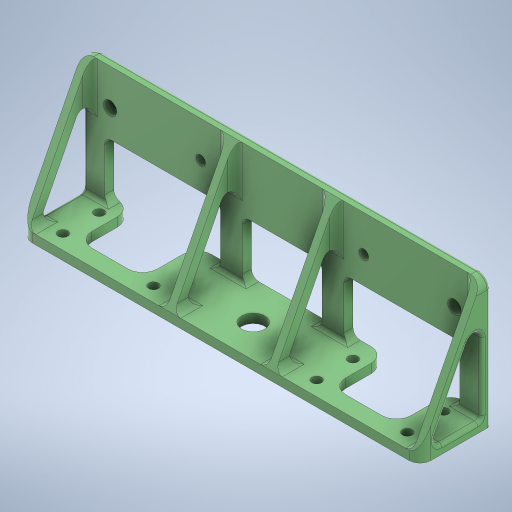
# Autodesk Inventor part: v3_realsense_mount
Saved by Autodesk Inventor 2024 (Build 280153000, 153)
## iProperties
Created: 2025-03-09
Part Number: v3_realsense_mount
Material: Generic
Document SubType Name: Modeling
Designer: Bruno
Density: 1 g/cm^3
Appearance: Default
Author: Bruno
Autodesk Inventor part; units mm, degrees
ref_plane "YZ Plane" through (0, 0, 0) normal (1, 0, 0) x (0, 1, 0)
ref_plane "XZ Plane" through (0, 0, 0) normal (0, 1, 0) x (-1, 0, 0)
sketch "Sketch1" plane through (0, 0, 0) normal (0, 1, 0) x (-1, 0, 0)
  line L0 (55, -9) -> (-55, -9)
  line L1 (-55, -9) -> (-55, 9)
  line L2 (-55, 9) -> (55, 9)
  line L3 (55, 9) -> (55, -9)
  line L4 (55, -9) -> (-55, 9)
  line L5 (55, 0) -> (-55, 0)
  line L6 (0, -9) -> (0, 9)
  circle A0 centre (0, 0) radius 3.2
  circle A1 centre (47.5, 5) radius 1.35
  circle A2 centre (22.5, 5) radius 1.35
  circle A3 centre (47.5, -5) radius 1.35
  circle A4 centre (22.5, -5) radius 1.35
  circle A5 centre (-47.5, 5) radius 1.35
  circle A6 centre (-22.5, 5) radius 1.35
  circle A7 centre (-47.5, -5) radius 1.35
  circle A8 centre (-22.5, -5) radius 1.35
  dimension "d0" = 18
  dimension "d1" = 110
  dimension "d2" = 6.4
  dimension "d3" = 2.7
  dimension "d4" = 2.7
  dimension "d5" = 45
  dimension "d6" = 95
  dimension "d7" = 10
  dimension "d8" = 10
  constraints: 14 end point, 9 centre point, 6 symmetric about line, 5 midpoint, 2 coincident, 2 parallel, 1 horizontal, 1 perpendicular, 6 other
  measures "d0" distance of L2.end L0.start
  measures "d1" distance of L1.end L2.end
  measures "d2" diameter of A0
  measures "d3" diameter of A1
  measures "d4" diameter of A2
  measures "d5" diameter of A2.centre L6
  measures "d6" diameter of A1.centre L6
  measures "d7" diameter of A2.centre L5
  measures "d8" diameter of A1.centre L5
extrude "Extrusion1" add sketch "Sketch1" along normal blind 2.5 contours L4 A4 A0 L5 L3 | L0 L6 A0 L4 A4 | L0 L1 L5 A0 L6 | L5 A0 L6 L2 L3 | L1 L4 A6 A0 L5 | L6 A0 L4 A6 L2
sketch "Sketch2" plane through (-55, 0, -9) normal (-1, 0, 0) x (0, 0, 1)
  line L0 (0, 0) -> (18, 0) projected
  line L1 (18, 0) -> (18, 2.5) projected
  line L2 (0, 2.5) -> (18, 2.5) projected
  line L3 (0, 0) -> (0, 2.5) projected
  line L4 (1, 0) -> (-1.5, 0)
  line L5 (-1.5, 0) -> (-1.5, 36)
  line L6 (-1.5, 36) -> (1, 36)
  line L7 (1, 36) -> (1, 0)
  point P0 (9, 0)
  point P1 (1, 2.5)
  dimension "d11" = 17
  dimension "d12" = 2.5
  dimension "d35" = 36
  constraints: 8 end point, 2 parallel, 1 horizontal, 1 perpendicular, 1 point on line
  measures "d11" distance between parallel lines of L7 L1
  measures "d12" distance of L5.end L6.end
  measures "d35" distance between parallel lines of L0 L6
extrude "Extrusion2" add sketch "Sketch2" against normal up to surface (110 mm away) contours L4 L5 L6 L7 L2 L3
sketch "Sketch3" plane through (-55, 2.5, -8) normal (0, 0, 1) x (1, 0, 0)
  line L0 (0, 33.5) -> (110, 33.5) projected
  line L1 (0, 0) -> (0, 33.5) projected
  line L2 (110, 0) -> (110, 33.5) projected
  line L3 (0, 23.5) -> (110, 23.5)
  circle A0 centre (7.5, 23.5) radius 1.85
  circle A1 centre (32.5, 23.5) radius 1.35
  line L4 (55, 33.5) -> (55, 1.216)
  circle A2 centre (102.5, 23.5) radius 1.85
  circle A3 centre (77.5, 23.5) radius 1.35
  line L5 (6, 16) -> (38, 16)
  line L6 (38, 16) -> (38, 0)
  line L7 (38, 0) -> (6, 0)
  line L8 (6, 0) -> (6, 16)
  line L9 (44, 16) -> (66, 16)
  line L10 (66, 16) -> (66, 0)
  line L11 (66, 0) -> (44, 0)
  line L12 (44, 0) -> (44, 16)
  line L13 (104, 16) -> (72, 16)
  line L14 (72, 16) -> (72, 0)
  line L15 (72, 0) -> (104, 0)
  line L16 (104, 0) -> (104, 16)
  line L17 (0, 0) -> (110, 0) projected
  point P0 (55, -2.5)
  point P1 (55, 23.5)
  point P2 (55, 16)
  dimension "d16" = 2.7
  dimension "d17" = 3.7
  dimension "d18" = 45
  dimension "d19" = 20
  dimension "d20" = 95
  dimension "d30" = 15
  dimension "d32" = 32
  dimension "d33" = 22
  dimension "d34" = 6
  constraints: 28 end point, 8 point on line, 6 symmetric about line, 4 centre point, 4 parallel, 3 midpoint, 3 perpendicular, 2 horizontal, 1 collinear, 1 vertical, 2 other
  measures "d16" diameter of A1
  measures "d17" diameter of A0
  measures "d18" diameter of A1.centre L4
  measures "d19" diameter of L0 L3
  measures "d20" diameter of A0.centre L4
  measures "d30" diameter of L5 L3
  measures "d32" distance of L5.start L5.end
  measures "d33" distance of L9.start L9.end
  measures "d34" distance between parallel lines of L12 L6
extrude "Extrusion3" cut sketch "Sketch3" against normal blind 10 contours A0 L3 | L3 A0 | A1 L3 | L3 A1 | A3 L3 | L3 A3 | L9 L10 L11 L12 | L8 L5 L6 L7 | A2 L3 | L3 A2 | L15 L14 L13 L16
sketch "Sketch4" plane through (-55, 0, 9) normal (-1, 0, 0) x (0, 0, 1)
  line L0 (-17, 2.5) -> (-17, 36) projected
  line L1 (-17, 2.5) -> (0, 2.5) projected
  line L2 (-17, 36) -> (0, 2.5)
  line L3 (-17, 30.4755) -> (-2.8035, 2.5)
  point P0 (-9, 0)
  dimension "d25" = 2.5
  constraints: 4 end point, 2 point on line, 1 parallel
  measures "d25" distance between parallel lines of L2 L3
extrude "Extrusion4" add sketch "Sketch4" against normal blind 2 contours L0 L2 L1 L3
pattern_linear "Rectangular Pattern1" count 2 spacing 40 along (1, 0, 0) of "Extrusion4"
ref_plane "Work Plane1" through (0, 0, -10.5) normal (-1, 0, 0) x (0, 0, 1)
mirror "Mirror1" about plane through (0, 0, -10.5) normal (-1, 0, 0) of "Extrusion4", "Rectangular Pattern1"
fillet "Fillet1" radius 2 32 edges at (-15, 33.2377, -8) (-13, 33.2377, -8) (13, 33.2377, -8) (15, 33.2377, -8) (-53, 33.2377, -8) (-54, 2.5, 6.1965) (-14, 2.5, 6.1965) (-17, 2.5, -9.25) (-17, 18.5, -9.25) (-49, 18.5, -9.25) (-49, 2.5, -9.25) (-11, 2.5, -9.25) (-11, 18.5, -9.25) (14, 2.5, 6.1965) (11, 2.5, -9.25) (11, 18.5, -9.25) (53, 33.2377, -8) (54, 2.5, 6.1965) (49, 18.5, -9.25) (49, 2.5, -9.25) (17, 18.5, -9.25) (17, 2.5, -9.25) (-13, 2.5, 7.5983) (15, 2.5, 7.5983) (13, 2.5, 7.5983) (-15, 2.5, 7.5983) (53, 2.5, 7.5983) (-53, 2.5, 7.5983) (-54, 30.4755, -8) (-14, 30.4755, -8) (54, 30.4755, -8) (14, 30.4755, -8)
fillet "Fillet2" radius 3 4 edges at (-55, 36, -9.25) (55, 36, -9.25) (55, 1.25, 9) (-55, 1.25, 9)
fillet "Fillet3" radius 1 25 edges at (-54.1213, 35.1213, -10.5) (0, 36, -10.5) (54.1213, 35.1213, -10.5) (55, 16.5, -10.5) (-55, 16.5, -10.5) (10, 2.5, -8) (14, 2.5, -8) (18, 2.5, -8) (-18, 2.5, -8) (-14, 2.5, -8) (-10, 2.5, -8) (-48, 2.5, -8) (-52, 2.5, -8) (48, 2.5, -8) (52, 2.5, -8) (55, 24.0598, -6.4653) (55, 14.2124, 0.2529) (55, 3.4536, 4.6432) (55, 2.5, -2.5306) (55, 12.3074, -8) (-55, 24.0598, -6.4653) (-55, 14.2124, 0.2529) (-55, 3.4536, 4.6432) (-55, 2.5, -2.5306) (-55, 12.3074, -8)
sketch "Sketch5" plane through (0, 2.5, 0) normal (0, 1, 0) x (1, 0, 0)
  line L0 (19, 10.5) -> (47, 10.5) projected
  line L1 (-47, 10.5) -> (-19, 10.5) projected
  line L2 (-9, 10.5) -> (9, 10.5) projected
  line L3 (0, 10.5) -> (0, -13.9758)
  circle A0 centre (-47.5, 5) radius 1.35 projected
  circle A1 centre (-22.5, 5) radius 1.35 projected
  line L4 (-47.5, 5) -> (-22.5, 5)
  line L5 (-35, 10.5) -> (-35, -12.5221)
  line L6 (-54, 10.5) -> (54, 10.5) projected
  line L7 (-44, 10.5) -> (-44, -4.5)
  line L8 (-44, -4.5) -> (-26, -4.5)
  line L9 (-26, -4.5) -> (-26, 10.5)
  line L10 (44, 10.5) -> (44, -4.5)
  line L11 (44, -4.5) -> (26, -4.5)
  line L12 (26, -4.5) -> (26, 10.5)
  point P0 (0, 0)
  point P1 (-35, 5)
  point P2 (-35, -4.5)
  dimension "d39" = 18
  dimension "d40" = 15
  constraints: 18 end point, 4 point on line, 4 symmetric about line, 3 midpoint, 3 perpendicular, 2 vertical, 1 horizontal, 2 other
  measures "d39" distance of L7.end L8.end
extrude "Extrusion5" cut sketch "Sketch5" against normal through all contours L0 L10 L11 L12 | L1 L5 L4 L7 | L1 L9 L4 L5 | L4 L5 L8 L7 | L4 L9 L8 L5
fillet "Fillet4" radius 4 8 edges at (-44, 1.25, -10.5) (-26, 1.25, -10.5) (-26, 1.25, 4.5) (-44, 1.25, 4.5) (26, 1.25, -10.5) (26, 1.25, 4.5) (44, 1.25, 4.5) (44, 1.25, -10.5)
body "Solid1"
